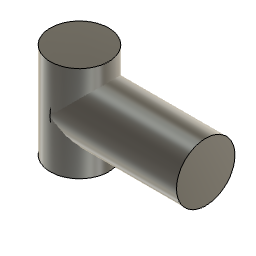
Arm 5 v1 (Autodesk Fusion 360 design; units mm, degrees)
Autodesk Fusion 360 part; units mm, degrees
cylinder "CylinderPrimitive1" add diameter 30 height 49 placed x (1, 0, 0) y (0, 1, 0) z (0, 0, 1) at (0, 0, 0) makes body 1
move_body "Move1" bodies 1 to x (1, 0, 0) y (0, 1, 0) z (0, 0, 1) at (0, 0, -24.5)
cylinder "CylinderPrimitive2" add diameter 30 height 50 placed x (0, 0, -1) y (0, 1, 0) z (1, 0, 0) at (0, -90, 0) separate body makes body 2
move_body "Move2" bodies 2 to x (1, 0, 0) y (0, 0.992546, 0.121869) z (0, -0.121869, 0.992546) at (20.062, 90.2453, 11.0964)
move_body "Move3" bodies 1 to x (1, 0, 0) y (0, 1, 0) z (0, 0, 1) at (-100, 0, 0)
move_body "Move4" bodies 2 to x (1, 0, 0) y (0, 1, 0) z (0, 0, 1) at (-1.5742, -1.1133, -6.1011)
move_body "Move5" bodies 2 to x (1, 0, 0) y (0, 1, 0) z (0, 0, 1) at (-18.5517, 0.1112, 6.3934)
move_body "Move6" bodies 1 to x (1, 0, 0) y (0, 1, 0) z (0, 0, 1) at (100, 0, 0)
extrude "Extrude1" add 1 faces at (49.9361, -0.4173, 1.6101) along direction (1, 0, 0) blind 15 on bodies 2 bodies 2
